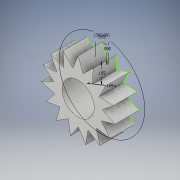
# Autodesk Inventor part: phonecasegearSMALL
Saved by Autodesk Inventor 2018.3 (Build 223284000, 284)
## iProperties
Created: 2019-03-12
Part Number: phonecasegearSMALL
Material: Generic
Document SubType Name: Modeling
Designer: F8PLTW
Density: 1 g/cm^3
Appearance: Default
Author: F8PLTW
Autodesk Inventor part; units mm, degrees
ref_plane "YZ Plane" through (0, 0, 0) normal (1, 0, 0) x (0, 1, 0)
ref_plane "XZ Plane" through (0, 0, 0) normal (0, 1, 0) x (-1, 0, 0)
ref_plane "XY Plane" through (0, 0, 0) normal (0, 0, 1) x (1, 0, 0)
sketch "Sketch1" plane through (0, 0, 0) normal (0, 0, 1) x (1, 0, 0)
  line L0 (-4.7131, 5.4277) -> (-2.9351, 5.4277)
  line L1 (-3.8241, 5.4277) -> (-3.8241, 7.7137) construction
  line L2 (-3.8241, 7.7137) -> (-2.9351, 5.4277)
  line L3 (-3.8241, 7.7137) -> (-4.7131, 5.4277)
  line L4 (-3.8241, 5.4277) -> (-3.8241, 2.7677) construction
  line L5 (-5.8358, 7.2861) -> (-4.0938, 5.5593)
  line L6 (-5.8358, 7.2861) -> (-5.7181, 4.8361)
  line L7 (-5.7181, 4.8361) -> (-4.0938, 5.5593)
  line L8 (-7.4997, 6.0772) -> (-5.206, 5.2082)
  line L9 (-7.4997, 6.0772) -> (-6.3957, 3.8869)
  line L10 (-6.3957, 3.8869) -> (-5.206, 5.2082)
  line L11 (-8.528, 4.2961) -> (-6.0792, 4.4352)
  line L12 (-8.528, 4.2961) -> (-6.6286, 2.7442)
  line L13 (-6.6286, 2.7442) -> (-6.0792, 4.4352)
  line L14 (-8.743, 2.2507) -> (-6.5624, 3.3738)
  line L15 (-8.743, 2.2507) -> (-6.3766, 1.6055)
  line L16 (-6.3766, 1.6055) -> (-6.5624, 3.3738)
  line L17 (-8.1074, 0.2947) -> (-6.5722, 2.2076)
  line L18 (-8.1074, 0.2947) -> (-5.6832, 0.6678)
  line L19 (-5.6832, 0.6678) -> (-6.5722, 2.2076)
  line L20 (-6.7313, -1.2337) -> (-6.1068, 1.1383)
  line L21 (-6.7313, -1.2337) -> (-4.6684, 0.0932)
  line L22 (-4.6684, 0.0932) -> (-6.1068, 1.1383)
  line L23 (-4.8524, -2.0702) -> (-5.2467, 0.3507)
  line L24 (-4.8524, -2.0702) -> (-3.5075, -0.019)
  line L25 (-3.5075, -0.019) -> (-5.2467, 0.3507)
  line L26 (-2.7957, -2.0702) -> (-4.1406, -0.019)
  line L27 (-2.7957, -2.0702) -> (-2.4014, 0.3507)
  line L28 (-2.4014, 0.3507) -> (-4.1406, -0.019)
  line L29 (-0.9169, -1.2337) -> (-2.9798, 0.0932)
  line L30 (-0.9169, -1.2337) -> (-1.5413, 1.1383)
  line L31 (-1.5413, 1.1383) -> (-2.9798, 0.0932)
  circle A0 centre (-3.8241, 2.7677) radius 2.9051
  circle A1 centre (-3.8241, 2.7677) radius 2.15
  line L32 (0.4593, 0.2947) -> (-1.9649, 0.6678)
  line L33 (0.4593, 0.2947) -> (-1.0759, 2.2076)
  line L34 (-1.0759, 2.2076) -> (-1.9649, 0.6678)
  line L35 (1.0948, 2.2507) -> (-1.2716, 1.6055)
  line L36 (1.0948, 2.2507) -> (-1.0857, 3.3738)
  line L37 (-1.0857, 3.3738) -> (-1.2716, 1.6055)
  line L38 (0.8799, 4.2961) -> (-1.0195, 2.7442)
  line L39 (0.8799, 4.2961) -> (-1.569, 4.4352)
  line L40 (-1.569, 4.4352) -> (-1.0195, 2.7442)
  line L41 (-0.1485, 6.0772) -> (-1.2524, 3.8869)
  line L42 (-0.1485, 6.0772) -> (-2.4422, 5.2082)
  line L43 (-2.4422, 5.2082) -> (-1.2524, 3.8869)
  line L44 (-1.8123, 7.2861) -> (-1.93, 4.8361)
  line L45 (-1.8123, 7.2861) -> (-3.5543, 5.5593)
  line L46 (-3.5543, 5.5593) -> (-1.93, 4.8361)
  point P0 (0, 0)
  point P1 (-4.906, 5.1977)
  point P2 (-5.8008, 4.5476)
  point P3 (-6.3539, 3.5897)
  point P4 (-6.4695, 2.4896)
  point P5 (-6.1277, 1.4377)
  point P6 (-5.3876, 0.6157)
  point P7 (-4.3771, 0.1658)
  point P8 (-3.271, 0.1658)
  point P9 (-2.2606, 0.6157)
  point P10 (-1.5204, 1.4377)
  point P11 (-1.1786, 2.4896)
  point P12 (-1.2943, 3.5897)
  point P13 (-1.8473, 4.5476)
  point P14 (-2.7421, 5.1977)
  dimension "d0" = 1.778
  dimension "d2" = 2.66
  dimension "d5" = 360
  dimension "d7" = 4.3
  dimension "d11" = 2.286
  constraints: 94 end point, 2 centre point, 2 coincident, 2 vertical, 1 horizontal, 1 midpoint, 106 other
  measures "d0" distance of L0.start L0.end
  measures "d2" distance of L1.start L4.end
  measures "d7" diameter of A1
  measures "d11" distance from line of L1.end L0
extrude "Extrusion2" add sketch "Sketch1" along normal blind 3.175 contours L3 A0 L5 L7 L0 | L0 L7 L10 L8 A0 L3 | L7 L5 A0 L45 L46 L0 | L0 L46 L43 L40 L37 L34 L31 L28 L25 L22 L19 L16 L13 L10 L7 | A0 L8 L6 L5 L3 | L3 L5 A0 | L46 L45 A0 L2 L0 | L0 L2 A0 L42 L43 L46 | L10 L13 L11 A0 L6 L7 | L7 L6 A0 L8 L10 | L3 L2 L45 A0 L5 | A0 L6 L8 | L46 L44 A0 L39 L40 L43 | L43 L42 A0 L44 L46 | L13 L16 L14 A0 L9 L10 | L10 L9 A0 L11 L13 | L45 L2 A0 | L6 A0 L11 L9 L8 | L43 L41 A0 L36 L37 L40 | L40 L39 A0 L41 L43 | L16 L19 L17 A0 L12 L13 | L13 L12 A0 L14 L16 | A0 L9 L11 | L40 L38 A0 L33 L34 L37 | L37 L36 A0 L38 L40 | A0 L14 L12 L11 L9 | L19 L22 L20 A0 L15 L16 | L16 L15 A0 L17 L19 | L37 L35 A0 L30 L31 L34 | L34 L33 A0 L35 L37 | A0 L12 L14 | A0 L17 L15 L14 L12 | L22 L25 L23 A0 L18 L19 | L19 L18 A0 L20 L22 | L34 L32 A0 L27 L28 L31 | L31 L30 A0 L32 L34 | A0 L15 L17 | A0 L20 L18 L17 L15 | L25 L28 L26 A0 L21 L22 | L22 L21 A0 L23 L25 | L31 L29 A0 L24 L25 L28 | L28 L27 A0 L29 L31 | A0 L18 L20 | A0 L23 L21 L20 L18 | L25 L24 A0 L26 L28 | L30 L32 A0 | L32 L30 L29 L27 A0 | A0 L21 L23 | A0 L26 L24 L23 L21 | L27 L29 A0 | L29 L27 L26 L24 A0 | A0 L24 L26
extrude "Extrusion3" add sketch "Sketch1" along normal blind 3.175 contours L46 L45 A0 L2 L0 | L0 L2 A0 L42 L43 L46 | L46 L44 A0 L39 L40 L43 | L43 L42 A0 L44 L46 | L45 L2 A0 | L2 L45 L44 L42 A0 | L43 L41 A0 L36 L37 L40 | L40 L39 A0 L41 L43 | L42 L44 A0 | L40 L38 A0 L33 L34 L37 | L37 L36 A0 L38 L40 | L44 L42 L41 L39 A0 | L39 L41 A0 | L37 L35 A0 L30 L31 L34 | L34 L33 A0 L35 L37 | L41 L39 L38 L36 A0 | L36 L38 A0 | L31 L30 A0 L32 L34 | L38 L36 L35 L33 A0 | L33 L35 A0 | L35 L33 L32 L30 A0 | L30 L32 A0
body "Solid2"
